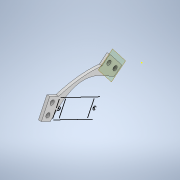
# Autodesk Inventor part: Part8
Saved by Autodesk Inventor 2020 (Build 240168000, 168)
## iProperties
Created: 2022-04-08
Part Number: Part8
Material: Generic
Document SubType Name: Modeling
Designer: Mic
Density: 1 g/cm^3
Appearance: Default
Author: Mic
Autodesk Inventor part; units mm, degrees
ref_plane "YZ Plane" through (0, 0, 0) normal (1, 0, 0) x (0, 1, 0)
ref_plane "XZ Plane" through (0, 0, 0) normal (0, 1, 0) x (-1, 0, 0)
ref_plane "XY Plane" through (0, 0, 0) normal (0, 0, 1) x (1, 0, 0)
ref_plane "Work Plane1" through (-16.2454, 8.6173, 20.7877) normal (-1, 0, 0) x (0, 0.7892, 0.6141)
sketch "Sketch1" plane through (-16.2454, 8.6173, 20.7877) normal (-1, 0, 0) x (0, 0.7892, 0.6141)
  circle A0 centre (-3.4689, 0) radius 1.5 projected
  circle A1 centre (3.4689, 0) radius 1.5 projected
  line L0 (6.8332, 3.5) -> (-6.8332, 3.5) projected
  line L1 (6.8332, -3.5) -> (6.8332, 3.5) projected
  line L2 (-6.8332, -3.5) -> (6.8332, -3.5) projected
  line L3 (-6.8332, 3.5) -> (-6.8332, -3.5) projected
  circle A2 centre (24.5746, -34.1307) radius 1.5 projected
  circle A3 centre (21.4751, -40.3376) radius 1.5 projected
  line L4 (23.1033, -44.9111) -> (29.2089, -32.6845) projected
  line L5 (16.8407, -41.7838) -> (23.1033, -44.9111) projected
  line L6 (22.9464, -29.5571) -> (16.8407, -41.7838) projected
  line L7 (29.2089, -32.6845) -> (22.9464, -29.5571) projected
  line L8 (22.9464, -29.5571) -> (16.8407, -13.9047) construction
  line L9 (16.8407, -13.9047) -> (6.8332, -3.5) construction
  spline S0 degree 2 poles (22.9464, -29.5571) (16.8407, -13.9047) (6.8332, -3.5) knots 1 1 1 2 2 2
  line L10 (16.8407, -41.7838) -> (18.1647, -31.1208) construction
  line L11 (18.1647, -31.1208) -> (21.4751, -11.5497) construction
  line L12 (21.4751, -11.5497) -> (4.0942, -7.8265) construction
  line L13 (4.0942, -7.8265) -> (-6.8332, -3.5) construction
  spline S1 degree 4 poles (16.8407, -41.7838) (18.1647, -31.1208) (21.4751, -11.5497) (4.0942, -7.8265) (-6.8332, -3.5) knots 1 1 1 1 1 2 2 2 2 2
  point P0 (-19.5675, 11.1132)
  constraints: 6 other
extrude "Extrusion1" add sketch "Sketch1" along normal blind 2
sketch "Sketch2" plane through (-16.2454, 8.6173, 20.7877) normal (1, 0, 0) x (0, 0.6141, -0.7892)
  arc A0 (-35.0948, 17.6868) -> (-34.1088, 18.1743) centre (-34.1796, 17.0766) ccw
  line L0 (-28.2545, 16.9384) -> (-37.6668, 12.2845)
  line L1 (-34.6395, 19.2477) -> (-30.4264, 21.3308)
  line L2 (-29.2877, 20.9456) -> (-15.8136, -6.3052)
  line L3 (-39.8387, 16.6769) -> (-35.6255, 18.7601)
  line L4 (-26.7498, -11.7126) -> (-40.2239, 15.5383)
  line L5 (-27.7829, -7.7054) -> (-18.3706, -3.0515)
  arc A1 (-20.9426, -8.4538) -> (-21.9287, -8.9413) centre (-21.8579, -7.8436) ccw
  point P0 (11.1132, -19.5675)
  constraints: 12 end point, 4 point on circle, 2 centre point, 26 other
body "Solid1"
